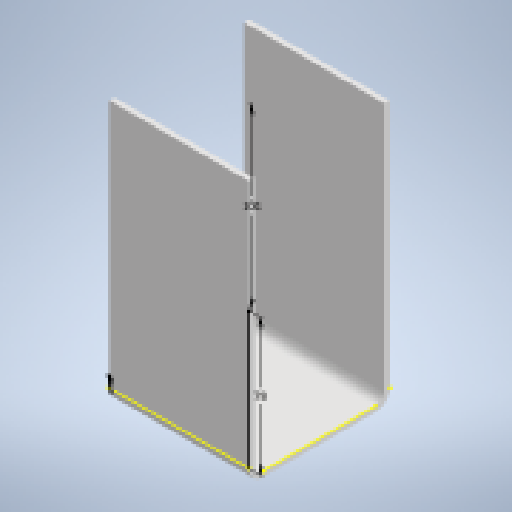
# Autodesk Inventor part: MSC 081 pillar 1
Saved by Autodesk Inventor 2025 (Build 290162010, 162A)
## iProperties
Created: 2024-06-25
Part Number: MSC 081 pillar 1
Material: Stainless Steel
Document SubType Name: Sheet Metal
Designer: admin
Density: 8 g/cm^3
Sheet Metal Rule: AISI304 3mm Die 32
Appearance: Default
Author: admin
Autodesk Inventor part; units mm, degrees
ref_plane "YZ Plane" through (0, 0, 0) normal (1, 0, 0) x (0, 1, 0)
ref_plane "XZ Plane" through (0, 0, 0) normal (0, 1, 0) x (-1, 0, 0)
ref_plane "XY Plane" through (0, 0, 0) normal (0, 0, 1) x (1, 0, 0)
sketch3d "3D Sketch1"
sketch "Sketch1" plane through (0, 0, 0) normal (0, 0, 1) x (1, 0, 0)
  line L0 (-40, 40) -> (40, 40)
  line L1 (40, 40) -> (40, -40)
  line L2 (40, -40) -> (-40, -40)
  line L3 (-40, -40) -> (-40, 40)
  line L4 (-40, 40) -> (40, -40) construction
  line L5 (40, 40) -> (-40, -40) construction
  point P0 (0, 0)
  dimension "d5" = 80
  measures "d5" distance of L1.end L2.end
extrude "Plate1" add sketch "Sketch1" along normal blind 3
sketch "Sketch2" plane through (40, -37, 0) normal (0, -1, 0) x (1, 0, 0)
  line L0 (-80, 0) -> (0, 0)
  line L1 (0, 0) -> (0, 200)
  line L2 (0, 200) -> (-80, 200)
  line L3 (-80, 200) -> (-80, 0)
  constraints: 6 end point, 1 horizontal, 1 perpendicular, 1 vertical
edge flange "Flange1" height 200 angle 90 thickness 3 bend radius 5 thickness toward (0, -1, 0) relief round relief width 3 relief depth 1.5 corner gap 5 corner form 0 edges at (0, -40, 3) (0, 40, 3) wall of the first edge with corners at (-40, -37, 0) (40, -37, 0) (40, -37, 200) (-40, -37, 200)
bend "Bend1"
corner "Corner1"
sketch3d "3D Sketch2"
ref_plane "Work Plane4" through (-40, -40, 28) normal (-0.5015382, -0.6617518, 0.5572647) x (0.7432941, 0, 0.6689647)
split "Split2" plane through (-40, -40, 28) removes the side toward (-0.5015382, -0.6617518, 0.5572647)
chamfer "Chamfer1" distance 2 angle 45 2 edges at (40, -38.5, 101.7813) (40, 38.5, 193.2188)
sketch "Sketch3" plane through (0, 0, 3) normal (0, 0, 1) x (1, 0, 0)
  line L0 (40, 32) -> (-40, 32) projected
  line L1 (-40, -32) -> (-40, 32) projected
  line L2 (-40, -32) -> (40, -32) projected
  line L3 (40, 32) -> (40, -32) projected
  line L4 (-40, -32) -> (-62, -32)
  line L5 (-62, -32) -> (-62, 32)
  line L6 (-62, 32) -> (-40, 32)
  circle A0 centre (-52, -22) radius 6.5
  circle A1 centre (-52, 22) radius 6.5
  line L7 (-40, 0) -> (-62, 0) construction
  point P0 (0, 0)
  dimension "d23" = 22
  dimension "d24" = 10
  dimension "d25" = 10
  dimension "d26" = 13
  constraints: 8 end point, 2 centre point, 2 midpoint, 2 perpendicular, 1 horizontal, 1 other
  measures "d23" distance of L1.start L4.end
  measures "d24" distance from line of L4 A0.centre
  measures "d25" distance from line of L5 A0.centre
  measures "d26" diameter of A0
extrude "Extrusion1" add sketch "Sketch3" against normal up to surface (3 mm away) contours L1 L4 L5 L6
mirror "Mirror1" about plane through (0, 0, 0) normal (1, 0, 0) of "Extrusion1"
fillet "Fillet1" radius 2 4 edges at (62, -32, 1.5) (62, 32, 1.5) (-62, 32, 1.5) (-62, -32, 1.5)
equation "\"d25\" = d24"
equation "\"d6\" = Thickness"
equation "\"d7\" = BendReliefWidth"
equation "\"d8\" = BendReliefDepth"
equation "\"d9\" = MinimumRemnant"
equation "\"d10\" = TransitionRadius"
equation "\"d13\" = BendRadius"
equation "\"d14\" = CornerReliefSize"
equation "\"d15\" = GapSize"
equation "\"d16\" = JacobiRadiusSize"
equation "\"BendReliefWidth\" = Thickness"
equation "\"BendReliefDepth\" = 0.5 * Thickness"
equation "\"CornerReliefSize\" = 4 * Thickness"
equation "\"MinimumRemnant\" = 2 * Thickness"
equation "\"TransitionRadius\" = BendRadius"
equation "\"JacobiRadiusSize\" = BendRadius"
equation "\"GapSize\" = Thickness"
equation "\"Thickness\" = 3"
equation "\"BendRadius\" = 5"
body "Solid1"
